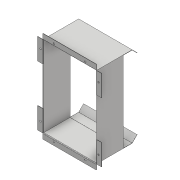
# Autodesk Inventor part: chimneyHousing
Saved by Autodesk Inventor 2017 (Build 210142000, 142)
## iProperties
Created: 2016-12-02
Part Number: chimneyHousing
Material: Generic
Document SubType Name: Modeling
Designer: krosie
Density: 1 g/cm^3
Appearance: Default
Author: krosie
Autodesk Inventor part; units mm, degrees
ref_plane "YZ Plane" through (0, 0, 0) normal (1, 0, 0) x (0, 1, 0)
ref_plane "XZ Plane" through (0, 0, 0) normal (0, 1, 0) x (-1, 0, 0)
ref_plane "XY Plane" through (0, 0, 0) normal (0, 0, 1) x (1, 0, 0)
sketch "Sketch1" plane through (0, 0, 0) normal (0, 1, 0) x (-1, 0, 0)
  line L0 (-75, 114) -> (75, 114)
  line L1 (75, 114) -> (75, -114)
  line L2 (75, -114) -> (-75, -114)
  line L3 (-75, -114) -> (-75, 114)
  line L4 (-75, 114) -> (75, -114) construction
  line L5 (75, 114) -> (-75, -114) construction
  line L6 (75.8, 114.8) -> (-75.8, 114.8)
  line L7 (-75.8, 114.8) -> (-75.8, -114.8)
  line L8 (-75.8, -114.8) -> (75.8, -114.8)
  line L9 (75.8, -114.8) -> (75.8, 114.8)
  point P0 (0, 0)
  dimension "d0" = 150
  dimension "d1" = 228
  dimension "d2" = 0.8
  constraints: 20 end point, 4 parallel, 2 midpoint, 2 perpendicular, 1 horizontal, 3 other
  measures "d0" distance of L1.end L2.end
  measures "d1" distance of L0.end L1.end
  measures "d2" distance between parallel lines of L0 L6
extrude "Extrusion1" add sketch "Sketch1" along normal blind 101.6
sketch "Sketch3" plane through (0, 0, 0) normal (0, -1, 0) x (1, 0, 0)
  line L0 (75.8, 114.8) -> (75.8, -114.8) projected
  line L1 (75.8, -114.8) -> (-75.8, -114.8) projected
  line L2 (75.8, 114.8) -> (75.8, -114.8)
  line L3 (75.8, -114.8) -> (90.8, -114.8)
  line L4 (90.8, -114.8) -> (90.8, 114.8)
  line L5 (90.8, 114.8) -> (75.8, 114.8)
  line L6 (75.8, -114.8) -> (-75.8, -114.8)
  line L7 (-75.8, -114.8) -> (-75.8, -129.8)
  line L8 (-75.8, -129.8) -> (75.8, -129.8)
  line L9 (75.8, -129.8) -> (75.8, -114.8)
  line L10 (-75.8, 114.8) -> (75.8, 114.8) projected
  line L11 (-75.8, -114.8) -> (-75.8, 114.8)
  line L12 (-75.8, 114.8) -> (-90.8, 114.8)
  line L13 (-90.8, 114.8) -> (-90.8, -114.8)
  line L14 (-90.8, -114.8) -> (-75.8, -114.8)
  line L15 (-75.8, 114.8) -> (75.8, 114.8)
  line L16 (75.8, 114.8) -> (75.8, 129.8)
  line L17 (75.8, 129.8) -> (-75.8, 129.8)
  line L18 (-75.8, 129.8) -> (-75.8, 114.8)
  point P0 (0, 0)
  dimension "d11" = 15
  dimension "d12" = 15
  dimension "d13" = 15
  dimension "d14" = 15
  constraints: 32 end point, 9 parallel, 4 perpendicular, 2 collinear, 1 vertical
  measures "d11" distance of L3.end L0.end
  measures "d12" distance of L7.end L1.end
  measures "d13" distance of L12.end L10.start
  measures "d14" distance of L16.end L0.start
extrude "Extrusion3" add sketch "Sketch3" against normal blind 0.8 contours L5 L4 L3 L0 | L10 L18 L17 L16 | L9 L8 L7 L1 | L11 L14 L13 L12
fillet "Fillet1" radius 2 4 edges at (75, 0, 0) (0, 0, -114) (-75, 0, 0) (0, 0, 114)
sketch "Sketch4" plane through (0, 0.8, 0) normal (0, 1, 0) x (1, 0, 0)
  line L0 (82.25, 120.65) -> (-82.25, 120.65) construction
  line L1 (-82.25, 120.65) -> (-82.25, -120.65) construction
  line L2 (-82.25, -120.65) -> (82.25, -120.65) construction
  line L3 (82.25, -120.65) -> (82.25, 120.65) construction
  line L4 (82.25, 120.65) -> (-82.25, -120.65) construction
  line L5 (-82.25, 120.65) -> (82.25, -120.65) construction
  line L6 (0, 0) -> (0, -60) construction
  line L7 (0, 0) -> (60, 0) construction
  point P0 (44.45, 120.65)
  point P1 (-44.45, 120.65)
  point P2 (-82.25, 88.9)
  point P3 (-82.25, 0)
  point P4 (-82.25, -88.9)
  point P5 (-44.45, -120.65)
  point P6 (44.45, -120.65)
  point P7 (82.25, -88.9)
  point P8 (82.25, 0)
  point P9 (82.25, 88.9)
  dimension "d18" = 164.5
  dimension "d19" = 241.3
  dimension "d20" = 88.9
  dimension "d21" = 60
  dimension "d22" = 90
  dimension "d23" = 88.9
  dimension "d24" = 88.9
  constraints: 16 end point, 8 point on line, 4 midpoint, 2 horizontal, 2 horizontal alignment, 2 parallel, 2 perpendicular, 2 vertical alignment, 1 symmetric about line, 1 vertical
  measures "d18" distance of L2.end L1.end
  measures "d19" distance of L1.end L0.end
  measures "d20" distance of point (-44.45, -120.65) point (44.45, -120.65)
  measures "d21" distance of L6.start L6.end
  measures "d22" angle of L6 L7
  measures "d23" distance of point (82.25, -88.9) point (82.25, 0)
  measures "d24" distance of point (82.25, 0) point (82.25, 88.9)
hole "Hole1" at (44.45, 0.8, -120.65) at (-44.45, 0.8, -120.65) at (-82.25, 0.8, -88.9) at (-82.25, 0.8, 0) at (-82.25, 0.8, 88.9) at (-44.45, 0.8, 120.65) at (44.45, 0.8, 120.65) at (82.25, 0.8, 88.9) at (82.25, 0.8, 0) at (82.25, 0.8, -88.9) direction (0, -1, 0) diameter 4.496 end through all clearance for "Flat Head Machine Screw (82)" size "#8" standard "Ansi Unified Screw Threads"
sketch "Sketch8" plane through (75.8, 101.6, 114.8) normal (1, 0, 0) x (0, 0, -1)
  line L0 (0.8, -99.6) -> (0.8, 0) projected
  line L1 (0.8, 0) -> (229, 0)
  line L2 (229, 0) -> (229, -25.4)
  line L3 (229, -25.4) -> (0.8, -25.4)
  line L4 (0.8, -25.4) -> (0.8, 0)
  point P0 (114.8, -101.6)
  dimension "d48" = 25.4
  constraints: 8 end point, 2 parallel, 1 perpendicular
  measures "d48" distance of L1.end L2.end
extrude "Extrusion7" cut sketch "Sketch8" against normal through all
sketch "Sketch9" plane through (75.8, 0.8, 114.8) normal (1, 0, 0) x (0, 0, -1)
  line L0 (0, 100.8) -> (14.1421, 114.9421)
  line L1 (0, 100.8) -> (20, 100.8) construction
  line L2 (14.5421, 114.5421) -> (0.8, 100.8)
  line L3 (14.1421, 114.9421) -> (14.5421, 114.5421)
  line L4 (229.6, 0) -> (229.6, 100.8) projected
  line L5 (229.6, 100.8) -> (215.4579, 114.9421)
  line L6 (229.6, 100.8) -> (249.6, 100.8) construction
  line L7 (215.1579, 114.6421) -> (229, 100.8)
  line L8 (229, 100.8) -> (229.6, 100.8) projected
  line L9 (229, 100.8) -> (229.6, 100.8)
  line L10 (215.4579, 114.9421) -> (215.1579, 114.6421)
  line L11 (0.8, 100.8) -> (0, 100.8) projected
  line L12 (0, 100.8) -> (0.8, 100.8)
  point P0 (114.8, -0.8)
  dimension "d51" = 20
  dimension "d52" = 45
  dimension "d53" = 20
  dimension "d54" = 135
  constraints: 20 end point, 3 perpendicular, 2 collinear, 2 equal length, 2 horizontal, 2 point on line, 1 coincident, 1 parallel
  measures "d51" distance of L0.start L0.end
  measures "d52" angle of L1 L0
  measures "d53" distance of L4.end L5.end
  measures "d54" angle of L6 L5
extrude "Extrusion8" add sketch "Sketch9" against normal up to surface (151.6 mm away)
sketch "Sketch10" plane through (0, 0.8, 0) normal (0, 1, 0) x (1, 0, 0)
  line L0 (75.8, 114.2) -> (75.8, -114) projected
  line L1 (-75.8, -114) -> (-75.8, 114.2) projected
  line L2 (-75.8, -114.8) -> (75.8, -114.8) projected
  line L3 (75.8, 114.8) -> (-75.8, 114.8) projected
  line L4 (90.8, -114.8) -> (90.8, 114.8) projected
  line L5 (90.8, -54.8) -> (75.8, -54.8)
  line L6 (75.8, -54.8) -> (75.8, 54.8)
  line L7 (75.8, 54.8) -> (90.8, 54.8)
  line L8 (90.8, 54.8) -> (90.8, -54.8)
  line L9 (90.8, 114.8) -> (75.8, 114.8) projected
  line L10 (75.8, -114.8) -> (90.8, -114.8) projected
  line L11 (0, 0) -> (0, 22) construction
  line L12 (-90.8, -54.8) -> (-75.8, -54.8)
  line L13 (-75.8, -54.8) -> (-75.8, 54.8)
  line L14 (-75.8, 54.8) -> (-90.8, 54.8)
  line L15 (-90.8, 54.8) -> (-90.8, -54.8)
  dimension "d57" = 60
  dimension "d58" = 60
  constraints: 18 end point, 4 symmetric about line, 2 parallel, 2 perpendicular, 2 point on line, 1 vertical
  measures "d57" distance between parallel lines of L9 L7
  measures "d58" distance between parallel lines of L10 L5
extrude "Extrusion9" cut sketch "Sketch10" against normal through all
body "Solid1"
